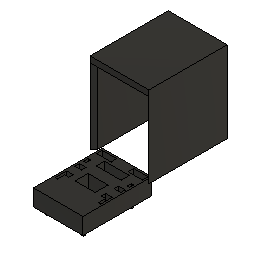
eth_usb_mount (Autodesk Fusion 360 design; units mm, degrees)
Autodesk Fusion 360 part; units mm, degrees
note: some values were not read from the file. Set by a fixed rule: which face or edge a step refers to.
sketch "rj45" plane through (0, 0, 0) normal (0, 0, 1) x (1, 0, 0)
  line L0 (35, 28) -> (54.4, 28)
  line L1 (54.4, 28) -> (54.4, 0.4)
  line L2 (54.4, 0.4) -> (35, 0.4)
  line L3 (35, 0.4) -> (35, 28)
  line L4 (44.7, 28) -> (44.7, -10)
  line L5 (35, 28) -> (41.1, 28)
  line L6 (41.1, 28) -> (41.1, 25.6)
  line L7 (41.1, 25.6) -> (35, 25.6)
  line L8 (35, 25.6) -> (35, 28)
  line L9 (35, 28) -> (35, 22)
  line L10 (35, 22) -> (36, 22)
  line L11 (36, 22) -> (36, 20.1)
  line L12 (36, 20.1) -> (35, 20.1)
  line L13 (35, 20.1) -> (35, 18.3)
  line L14 (35, 18.3) -> (37.8, 18.3)
  line L15 (37.8, 18.3) -> (37.8, 16.4)
  line L16 (37.8, 16.4) -> (35, 16.4)
  line L17 (35, 16.4) -> (35, 12.9)
  line L18 (35, 12.9) -> (37.8, 12.9)
  line L19 (37.8, 12.9) -> (37.8, 11)
  line L20 (37.8, 11) -> (35, 11)
  line L21 (36, 11) -> (36, 8)
  line L22 (36, 8) -> (35, 8)
  line L23 (54.4, 22) -> (53.4, 22)
  line L24 (53.4, 22) -> (53.4, 20.1)
  line L25 (53.4, 20.1) -> (54.4, 20.1)
  line L26 (54.4, 28) -> (48.3, 28)
  line L27 (48.3, 28) -> (48.3, 25.6)
  line L28 (54.4, 25.6) -> (54.4, 28)
  line L29 (48.3, 25.6) -> (54.4, 25.6)
  line L30 (54.4, 18.3) -> (51.6, 18.3)
  line L31 (51.6, 18.3) -> (51.6, 16.4)
  line L32 (51.6, 16.4) -> (54.4, 16.4)
  line L33 (54.4, 12.9) -> (51.6, 12.9)
  line L34 (51.6, 12.9) -> (51.6, 11)
  line L35 (51.6, 11) -> (54.4, 11)
  line L36 (53.4, 8) -> (54.4, 8)
  line L37 (53.4, 11) -> (53.4, 8)
  line L38 (44.7, 28) -> (44.7, 24.5)
  line L39 (49.95, 24.5) -> (39.45, 24.5)
  line L40 (39.45, 24.5) -> (39.45, 21)
  line L41 (39.45, 21) -> (49.95, 21)
  line L42 (49.95, 21) -> (49.95, 24.5)
  line L43 (44.7, 21) -> (44.7, 16.5)
  line L44 (48.95, 16.5) -> (40.45, 16.5)
  line L45 (40.45, 16.5) -> (40.45, 11)
  line L46 (48.95, 16.5) -> (48.95, 11)
  line L47 (48.95, 11) -> (40.45, 11)
  line L48 (55.2, 28.8) -> (55.2, -0.4)
  line L49 (55.2, -0.4) -> (34.2, -0.4)
  line L50 (34.2, -0.4) -> (34.2, 28.8)
  line L51 (34.2, 28.8) -> (55.2, 28.8)
  line L52 (56.2, -1.4) -> (33.2, -1.4)
  line L53 (33.2, -1.4) -> (33.2, 29.8)
  line L54 (33.2, 29.8) -> (56.2, 29.8)
  line L55 (56.2, 29.8) -> (56.2, -1.4)
  line L56 (57.2, -2.4) -> (32.2, -2.4)
  line L57 (32.2, -2.4) -> (32.2, 30.8)
  line L58 (32.2, 30.8) -> (57.2, 30.8)
  line L59 (57.2, 30.8) -> (57.2, -2.4)
  dimension "d1" = 27.6
  dimension "d2" = 19.4
  dimension "d3" = 6.1
  dimension "d4" = 2.4
  dimension "d5" = 1.9
  dimension "d6" = 1.8
  dimension "d7" = 2.8
  dimension "d8" = 1.9
  dimension "d9" = 3.5
  dimension "d10" = 2.8
  dimension "d11" = 3.5
  dimension "d12" = 10.5
  dimension "d13" = 3.5
  dimension "d14" = 4.5
  dimension "d15" = 8.5
  dimension "d16" = -0.8
  dimension "d17" = -1
  dimension "d18" = -1
  constraint horizontal L0
  constraint vertical L1
  constraint horizontal L2
  constraint vertical L3
  constraint midpoint L0 L4.start
  constraint perpendicular L2 L4
  constraint horizontal L5
  constraint vertical L6
  constraint horizontal L7
  constraint vertical L8
  constraint coincident L3 L9.end
  constraint perpendicular L3 L10
  constraint perpendicular L10 L11
  constraint coincident L3 L12.end
  constraint perpendicular L11 L12
  constraint perpendicular L12 L13
  constraint perpendicular L3 L14
  constraint perpendicular L14 L15
  constraint coincident L3 L16.end
  constraint perpendicular L3 L16
  constraint perpendicular L16 L17
  constraint perpendicular L17 L18
  constraint perpendicular L18 L19
  constraint coincident L3 L20.end
  constraint perpendicular L3 L20
  constraint coincident L20 L21.start
  constraint perpendicular L20 L21
  constraint coincident L3 L22.end
  constraint perpendicular L3 L22
  constraint symmetric L0.start L4 L0.end
  constraint symmetric L4 L5.end L26.end
  constraint symmetric L4 L6.end L27.end
  constraint symmetric L4 L7.end L28.start
  constraint symmetric L4 L9.end L23.start
  constraint symmetric L4 L10.end L23.end
  constraint symmetric L4 L11.end L24.end
  constraint symmetric L4 L12.end L25.end
  constraint symmetric L4 L13.end L30.start
  constraint symmetric L4 L14.end L30.end
  constraint symmetric L4 L15.end L31.end
  constraint symmetric L4 L16.end L32.end
  constraint symmetric L4 L17.end L33.start
  constraint symmetric L4 L18.end L33.end
  constraint symmetric L4 L19.end L34.end
  constraint symmetric L4 L20.end L35.end
  constraint symmetric L4 L21.start L37.start
  constraint symmetric L4 L21.end L36.start
  constraint symmetric L4 L22.end L36.end
  constraint perpendicular L0 L38
  constraint midpoint L38.end L39
  constraint perpendicular L4 L39
  constraint perpendicular L39 L40
  constraint perpendicular L40 L41
  constraint perpendicular L39 L42
  constraint midpoint L41 L43.start
  constraint perpendicular L41 L43
  constraint midpoint L43.end L44
  constraint perpendicular L43 L44
  constraint perpendicular L44 L45
  constraint perpendicular L44 L46
  constraint perpendicular L45 L47
  measures "d1" distance of L0.start L2.end
  measures "d2" distance of L0.start L0.end
  measures "d3" distance of L0.start L5.end
  measures "d4" distance of L0.start L7.end
  measures "d5" distance of L10.end L11.end
  measures "d6" distance of L12.end L13.end
  measures "d7" distance of L13.end L14.end
  measures "d8" distance of L14.end L15.end
  measures "d9" distance of L16.end L17.end
  measures "d10" distance of L17.end L18.end
  measures "d11" distance of L4.start L38.end
  measures "d12" distance of L39.start L39.end
  measures "d13" distance of L39.end L40.end
  measures "d14" distance of L43.start L43.end
  measures "d15" distance of L44.start L44.end
extrude "Extrude1" add sketch "rj45" against normal blind 7 contours L0 L3 L5 L6 L7 L8 L9 | L0 L2 L3 L4 L6 L7 L9 L10 L11 L12 L13 L14 L15 L16 L17 L18 L19 L20 L21 L22 L38 L39 L40 L41 L43 L44 L45 L47 | L0 L1 L2 L4 L23 L24 L25 L27 L29 L30 L31 L32 L33 L34 L35 L36 L37 L38 L39 L41 L42 L43 L44 L46 L47 | L3 L10 L11 L12 | L0 L1 L26 L27 L28 L29 | L4 L39 L41 L42 | L4 L39 L40 L41 | L3 L14 L15 L16 | L4 L44 L46 L47 | L4 L44 L45 L47 | L1 L23 L24 L25 | L3 L18 L19 L20 | L3 L20 L21 L22 | L1 L30 L31 L32 | L1 L35 L36 L37 | L1 L33 L34 L35 | L48 L49 L50 L51 | L52 L53 L54 L55 makes body 1
extrude "Extrude2" cut sketch "rj45" against normal blind 25 contours L52 L53 L54 L55 bodies 1
extrude "Extrude3" cut sketch "rj45" against normal blind 16 contours L0 L3 L5 L6 L7 L8 L9 | L3 L10 L11 L12 | L0 L1 L26 L27 L28 L29 | L4 L39 L41 L42 | L4 L39 L40 L41 | L3 L14 L15 L16 | L4 L44 L46 L47 | L4 L44 L45 L47 | L1 L23 L24 L25 | L3 L18 L19 L20 | L3 L20 L21 L22 | L1 L30 L31 L32 | L1 L35 L36 L37 | L1 L33 L34 L35 bodies 1
extrude "Extrude4" add sketch "rj45" along normal blind 32 separate body contours L52 L53 L54 L55 | L56 L57 L58 L59 makes body 2
move_face "OffsetFaces1" offset -9 2 faces at (51.7, -0.4, 10.6667) (41.2, -0.4, 10.6667) on bodies 2
extrude "Extrude5" add 1 faces at (32.8667, 19.0667, 32) along direction (0, 0, 1) blind 2.5 separate body on bodies 2 makes body 3
move_face "OffsetFaces2" offset 11 3 faces at (34.2, 8, 33.6667) (41.2, 28.8, 32.8333) (55.2, 18.4, 33.6667) on bodies 3
chamfer "Chamfer1" distance 2 angle 45 2 edges at (34.2, -2.4, 16) (55.2, -2.4, 16) tangent chain off on bodies 2
move_face "OffsetFaces3" offset -0.5 3 faces at (34.2, 9.3331, 21.3333) (41.2, 28.8, 10.6667) (55.2, 19.0665, 10.6667) on bodies 2
sketch "Sketch2" plane through (0, 0, -7) normal (0, 0, -1) x (1, 0, 0)
  line L0 (34.2, -28.8) -> (55.2, -28.8)
  line L1 (55.2, -28.8) -> (55.2, 0.4)
  line L2 (55.2, 0.4) -> (34.2, 0.4)
  line L3 (34.2, 0.4) -> (34.2, -28.8)
  line L4 (53.4, -22) -> (53.4, -20.1)
  line L5 (53.4, -20.1) -> (54.4, -20.1)
  line L6 (54.4, -20.1) -> (54.4, -22)
  line L7 (54.4, -22) -> (53.4, -22)
  line L8 (37.8, -18.3) -> (35, -18.3)
  line L9 (35, -18.3) -> (35, -16.4)
  line L10 (35, -16.4) -> (37.8, -16.4)
  line L11 (37.8, -16.4) -> (37.8, -18.3)
  line L12 (49.95, -24.5) -> (39.45, -24.5)
  line L13 (39.45, -24.5) -> (39.45, -21)
  line L14 (39.45, -21) -> (49.95, -21)
  line L15 (49.95, -21) -> (49.95, -24.5)
  line L16 (35, -28) -> (35, -25.6)
  line L17 (35, -25.6) -> (41.1, -25.6)
  line L18 (41.1, -25.6) -> (41.1, -28)
  line L19 (41.1, -28) -> (35, -28)
  line L20 (36, -11) -> (37.8, -11)
  line L21 (37.8, -11) -> (37.8, -12.9)
  line L22 (37.8, -12.9) -> (35, -12.9)
  line L23 (35, -12.9) -> (35, -8)
  line L24 (35, -8) -> (36, -8)
  line L25 (36, -8) -> (36, -11)
  line L26 (51.6, -18.3) -> (51.6, -16.4)
  line L27 (51.6, -16.4) -> (54.4, -16.4)
  line L28 (54.4, -16.4) -> (54.4, -18.3)
  line L29 (54.4, -18.3) -> (51.6, -18.3)
  line L30 (36, -22) -> (35, -22)
  line L31 (35, -22) -> (35, -20.1)
  line L32 (35, -20.1) -> (36, -20.1)
  line L33 (36, -20.1) -> (36, -22)
  line L34 (40.45, -16.5) -> (40.45, -11)
  line L35 (40.45, -11) -> (48.95, -11)
  line L36 (48.95, -11) -> (48.95, -16.5)
  line L37 (48.95, -16.5) -> (40.45, -16.5)
  line L38 (54.4, -25.6) -> (54.4, -28)
  line L39 (54.4, -28) -> (48.3, -28)
  line L40 (48.3, -28) -> (48.3, -25.6)
  line L41 (48.3, -25.6) -> (54.4, -25.6)
  line L42 (51.6, -12.9) -> (51.6, -11)
  line L43 (51.6, -11) -> (53.4, -11)
  line L44 (53.4, -11) -> (53.4, -8)
  line L45 (53.4, -8) -> (54.4, -8)
  line L46 (54.4, -8) -> (54.4, -12.9)
  line L47 (54.4, -12.9) -> (51.6, -12.9)
  line L48 (34.2, 0.4) -> (37.2, 0.4)
  line L49 (37.2, 0.4) -> (37.2, -2.6)
  line L50 (37.2, -2.6) -> (34.2, -2.6)
  line L51 (34.2, -2.6) -> (34.2, 0.4)
  circle A0 centre (37.2, -2.6) radius 0.7
  circle A1 centre (52.44, -2.6) radius 0.7
  circle A2 centre (37.2, -22.92) radius 0.7
  circle A3 centre (52.44, -22.92) radius 0.7
  dimension "d33" = 3
  dimension "d34" = 3
  dimension "d35" = 1.4
  dimension "d38" = 15.24
  dimension "d39" = -20.32
  constraint horizontal L48
  constraint vertical L49
  constraint horizontal L50
  constraint vertical L51
  constraint coincident L2.end L3.start
  constraint coincident L49.end L50.start
  measures "d33" distance of L2.end L48.end
  measures "d34" distance of L2.end L50.end
  measures "d35" diameter of A0
extrude "Extrude6" add sketch "Sketch2" along normal blind 2.6 contours L49 L50 A0 | L49 L50 A0 | A1 | A2 | A3 bodies 1
combine "Combine1" operation add target body 2 tool bodies 3
move_body "Move1" bodies 2 to x (1, 0, 0) y (0, 1, 0) z (0, 0, 1) at (0, 28, 0)
equation "d38 = 2.54 mm * 6"
equation "d39 = ( -2.54 * 8 ) * 1 mm"
named bodies: "position_mount", "protect_housing"
